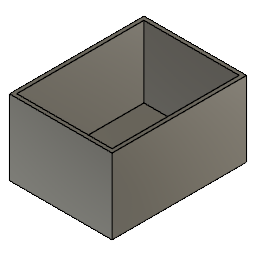
main_enclosure_12_cores (Autodesk Fusion 360 design; units mm, degrees)
Autodesk Fusion 360 part; units mm, degrees
sketch "Sketch1" plane through (0, 0, 0) normal (0, 0, 1) x (1, 0, 0)
  line L0 (27.3, 35.75) -> (-27.3, 35.75)
  line L1 (-27.3, 35.75) -> (-27.3, -35.75)
  line L2 (-27.3, -35.75) -> (27.3, -35.75)
  line L3 (27.3, -35.75) -> (27.3, 35.75)
  line L4 (27.3, 35.75) -> (-27.3, -35.75) construction
  line L5 (-27.3, 35.75) -> (27.3, -35.75) construction
  dimension "d1" = 54.6
  dimension "d2" = 71.5
  constraint perpendicular L0 L1
  constraint parallel L0 L2
  constraint parallel L1 L3
  constraint horizontal L0
  constraint coincident L4 origin
  constraint coincident L5 origin
  measures "d1" distance of L1.end L2.end
  measures "d2" distance of L0.end L1.end
extrude "Extrude1" add sketch "Sketch1" along normal blind 40
sketch "Sketch2" plane through (0, 0, 40) normal (0, 0, 1) x (-1, 0, 0)
  line L0 (-27.3, 35.75) -> (-27.3, -35.75)
  line L1 (-27.3, -35.75) -> (27.3, -35.75)
  line L2 (27.3, -35.75) -> (27.3, 35.75)
  line L3 (27.3, 35.75) -> (-27.3, 35.75)
  line L4 (-25.3, -33.75) -> (25.3, -33.75)
  line L5 (25.3, -33.75) -> (25.3, 33.75)
  line L6 (25.3, 33.75) -> (-25.3, 33.75)
  line L7 (-25.3, 33.75) -> (-25.3, -33.75)
  line L8 (-25.3, -33.75) -> (25.3, 33.75) construction
  line L9 (25.3, -33.75) -> (-25.3, 33.75) construction
  dimension "d5" = 50.6
  dimension "d6" = 67.5
  constraint perpendicular L4 L5
  constraint parallel L4 L6
  constraint parallel L5 L7
  constraint horizontal L4
  constraint coincident L8 origin
  constraint coincident L9 origin
  measures "d5" distance of L5.end L6.end
  measures "d6" distance of L4.end L5.end
extrude "Extrude2" cut sketch "Sketch2" against normal blind 38 contours L4 L5 L6 L7
sketch "Sketch3" plane through (0, 0, 2) normal (0, 0, 1) x (-1, 0, 0)
  line L0 (-25.3, 33.75) -> (-25.3, -33.75)
  line L1 (-25.3, -33.75) -> (25.3, -33.75)
  line L2 (25.3, -33.75) -> (25.3, 33.75)
  line L3 (25.3, 33.75) -> (-25.3, 33.75)
  line L4 (20, 20) -> (14, 20)
  line L5 (14, 20) -> (14, 30.3)
  line L6 (14, 30.3) -> (20, 30.3)
  line L7 (20, 30.3) -> (20, 20)
  dimension "d9" = 6
  dimension "d10" = 10.3
  constraint horizontal L4
  constraint vertical L5
  constraint horizontal L6
  constraint vertical L7
  measures "d9" distance of L4.start L4.end
  measures "d10" distance of L4.start L6.end
extrude "Extrude3" cut sketch "Sketch3" against normal blind 2 contours L4 L5 L6 L7
